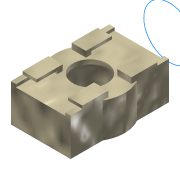
# Autodesk Inventor part: PI_holder
Saved by Autodesk Inventor 2014 (Build 180170000, 170)
## iProperties
Created: 2016-07-07
Part Number: PI_holder
Material: Generic
Document SubType Name: Modeling
Designer: Camilo
Density: 1 g/cm^3
Appearance: Fine - Cream
Author: Camilo
Autodesk Inventor part; units mm, degrees
ref_plane "YZ Plane" through (0, 0, 0) normal (1, 0, 0) x (0, 1, 0)
ref_plane "XZ Plane" through (0, 0, 0) normal (0, 1, 0) x (-1, 0, 0)
ref_plane "XY Plane" through (0, 0, 0) normal (0, 0, 1) x (1, 0, 0)
sketch "Sketch1" plane through (0, 0, 0) normal (0, 0, 1) x (1, 0, 0)
  circle A0 centre (0, 0) radius 7.925 projected
  circle A1 centre (0, 0) radius 8.425
  point P0 (0, 0)
  dimension "d0" = 0.5
  constraints: 1 centre point
  measures "d0" radial gap between concentric circles of A1 A0
extrude "Extrusion1" add sketch "Sketch1" along normal blind 1.5 contours A0 | A1
sketch "Sketch2" plane through (0, 0, 1.5) normal (0, 0, 1) x (1, 0, 0)
  circle A0 centre (0, 0) radius 8.425 projected
  circle A1 centre (0, 0) radius 11.425
  dimension "d3" = 3
  constraints: 1 centre point
  measures "d3" radial gap between concentric circles of A1 A0
extrude "Extrusion2" add sketch "Sketch2" against normal blind 12
sketch "Sketch3" plane through (0, 0, 1.5) normal (0, 0, 1) x (1, 0, 0)
  circle A0 centre (0, 0) radius 6.94 projected
  circle A1 centre (0, 0) radius 5.94
  dimension "d6" = 1
  constraints: 1 centre point
  measures "d6" radial gap between concentric circles of A0 A1
extrude "Extrusion3" cut sketch "Sketch3" against normal through all contours A1
sketch "Sketch4" plane through (0, 0, 1.5) normal (0, 0, 1) x (1, 0, 0)
  line L0 (-8.355, 16.96) -> (-8.355, 7.9) projected
  line L1 (8.355, 7.9) -> (8.355, 16.96) projected
  line L2 (-10.355, 17.0459) -> (10.355, 17.0459)
  line L3 (10.355, 17.0459) -> (10.355, 5.9)
  line L4 (-10.355, 5.9) -> (-10.355, 17.0459)
  circle A0 centre (0, 0) radius 10.575 projected
  line L5 (-8.7761, 5.9) -> (-10.355, 5.9)
  line L6 (10.355, 5.9) -> (8.7761, 5.9)
  arc A1 (8.7761, 5.9) -> (-8.7761, 5.9) centre (0, 0) ccw
  constraints: 10 end point, 4 point on circle, 1 centre point
extrude "Extrusion4" add sketch "Sketch4" against normal up to surface (12 mm away) contours L2 L3 L6 A0 L5 L4
sketch "Sketch5" plane through (0, 0, 1.5) normal (0, 0, 1) x (1, 0, 0)
  line L0 (10.355, 17.0459) -> (-10.355, 17.0459) projected
  line L1 (-8.355, 16.96) -> (-8.355, 7.9) projected
  line L2 (8.355, 7.9) -> (8.355, 16.96) projected
  line L3 (-6.395, 5.94) -> (6.395, 5.94) projected
  line L4 (-8.555, 17.0459) -> (-8.555, 7.9)
  line L5 (-8.555, 7.9) -> (-8.555, 5.94)
  line L6 (-8.555, 5.94) -> (-8.555, 5.84)
  line L7 (-8.555, 5.84) -> (-5.4211, 5.84)
  line L8 (-5.4211, 5.84) -> (-5.4211, 4.0009)
  line L9 (-5.4211, 4.0009) -> (-10.355, 4.0009)
  line L10 (-10.355, 4.0009) -> (-10.355, 17.0459)
  line L11 (-10.355, 17.0459) -> (-8.555, 17.0459)
  dimension "d12" = 0.2
  dimension "d13" = 0.1
  constraints: 16 end point, 1 point on line
  measures "d12" distance between parallel lines of L4 L1
  measures "d13" distance between parallel lines of L3 L7
extrude "Extrusion5" add sketch "Sketch5" along normal blind 1
sketch "Sketch6" plane through (0, 0, 2.5) normal (0, 0, 1) x (1, 0, 0)
  line L0 (-10.355, 4.0009) -> (-5.4211, 4.0009)
  line L1 (-5.4211, 4.0009) -> (-5.4211, 13.0009)
  line L2 (-5.4211, 13.0009) -> (-10.355, 13.0009)
  line L3 (-10.355, 13.0009) -> (-10.355, 4.0009)
  point P0 (0, 0)
  dimension "d18" = 9
  constraints: 8 end point, 2 horizontal, 1 vertical
  measures "d18" distance of L0.end L1.end
extrude "Extrusion6" add sketch "Sketch6" along normal blind 1
mirror "Mirror1" about plane through (0, 0, 0) normal (1, 0, 0) of "Extrusion5", "Extrusion6"
mirror "Mirror2" about plane through (0, 0, 0) normal (0, 1, 0) of "Extrusion5", "Extrusion6", "Mirror1", "Extrusion4"
body "Solid1"
